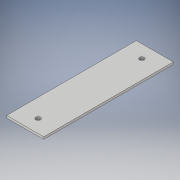
# Autodesk Inventor part: BAGMotor Beam
Saved by Autodesk Inventor 2017 (Build 210142000, 142)
## iProperties
Created: 2016-09-26
Part Number: BAGMotor Beam
Material: Generic
Document SubType Name: Modeling
Designer: Hanson
Density: 1 g/cm^3
Appearance: Default
Author: Hanson
Autodesk Inventor part; units mm, degrees
ref_plane "YZ Plane" through (0, 0, 0) normal (1, 0, 0) x (0, 1, 0)
ref_plane "XZ Plane" through (0, 0, 0) normal (0, 1, 0) x (-1, 0, 0)
ref_plane "XY Plane" through (0, 0, 0) normal (0, 0, 1) x (1, 0, 0)
sketch "Sketch1" plane through (0, 0, 0) normal (0, 1, 0) x (-1, 0, 0)
  line L0 (0, 0) -> (-25.4, 0)
  line L1 (-25.4, 0) -> (-25.4, -178.054)
  line L2 (-25.4, -178.054) -> (0, -178.054)
  line L3 (0, -178.054) -> (0, 0)
  dimension "d0" = 25.4
  dimension "d1" = 178.054
  constraints: 8 end point, 2 parallel, 1 horizontal, 1 perpendicular
  measures "d0" distance of L2.end L1.end
  measures "d1" distance of L0.end L1.end
extrude "Extrusion1" add sketch "Sketch1" along normal blind 3.175
sketch "Sketch2" plane through (0, 3.175, 0) normal (0, 1, 0) x (1, 0, 0)
  line L0 (0, 178.054) -> (0, 0) projected
  line L1 (0, 0) -> (25.4, 0) projected
  point P0 (12.7, 17.78)
  dimension "d4" = 12.7
  dimension "d5" = 17.78
  measures "d4" distance from line of L0 point (12.7, 17.78)
  measures "d5" distance from line of L1 point (12.7, 17.78)
hole "Hole1" at (12.7, 3.175, -17.78) direction (0, -1, 0) diameter 6.35 end through all
ref_plane "Work Plane1" through (25.4, 0, -89.027) normal (0, 0, -1) x (-1, 0, 0)
mirror "Mirror1" about plane through (25.4, 0, -89.027) normal (0, 0, -1) of "Hole1"
sketch "Sketch3" plane through (25.4, 0, 0) normal (1, 0, 0) x (0, 0, -1)
  line L0 (0, 3.175) -> (178.054, 3.175) projected
  line L1 (0, 0) -> (178.054, 0) projected
  line L2 (0, 3.175) -> (178.054, 3.175)
  line L3 (178.054, 3.175) -> (178.054, 0)
  line L4 (178.054, 0) -> (0, 0)
  line L5 (0, 0) -> (0, 3.175)
  constraints: 8 end point, 2 parallel, 1 horizontal, 1 perpendicular
extrude "Extrusion2" add sketch "Sketch3" along normal blind 12.7
sketch "Sketch4" plane through (0, 0, -178.054) normal (-1, 0, 0) x (0, 0, 1)
  line L0 (0, 0) -> (0, 3.175) projected
  line L1 (178.054, 0) -> (0, 0)
  line L2 (0, 0) -> (0, 3.175)
  line L3 (0, 3.175) -> (178.054, 3.175)
  line L4 (178.054, 3.175) -> (178.054, 0)
  constraints: 8 end point, 2 parallel, 1 horizontal, 1 perpendicular
extrude "Extrusion3" add sketch "Sketch4" along normal blind 12.7
body "Solid1"
